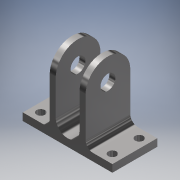
# Autodesk Inventor part: Custom Pneumatic Support
Saved by Autodesk Inventor 2019.4 (Build 234330000, 330)
## iProperties
Created: 2020-01-02
Part Number: Custom Pneumatic Support
Material: Stainless Steel
Document SubType Name: Modeling
Designer: Mark
Mass: 154.479 g
Surface Area: 101.01 cm^2
Volume: 19.3099 cm^3
Density: 8 g/cm^3
Appearance: Semi-Polished
Author: Mark
Autodesk Inventor part; units mm, degrees
ref_plane "YZ Plane" through (0, 0, 0) normal (1, 0, 0) x (0, 1, 0)
ref_plane "XZ Plane" through (0, 0, 0) normal (0, 1, 0) x (-1, 0, 0)
ref_plane "XY Plane" through (0, 0, 0) normal (0, 0, 1) x (1, 0, 0)
sketch "Sketch1" plane through (0, 0, 0) normal (0, 1, 0) x (-1, 0, 0)
  line L0 (-30, 15) -> (30, 15)
  line L1 (30, 15) -> (30, -15)
  line L2 (30, -15) -> (-30, -15)
  line L3 (-30, -15) -> (-30, 15)
  line L4 (-30, 15) -> (30, -15) construction
  line L5 (30, 15) -> (-30, -15) construction
  circle A0 centre (24, -9) radius 2.75
  circle A1 centre (24, 9) radius 2.75
  circle A2 centre (-24, 9) radius 2.75
  circle A3 centre (-24, -9) radius 2.75
  point P0 (0, 0)
  dimension "d0" = 60
  dimension "d1" = 30
  dimension "d2" = 5.5
  dimension "d3" = 5.5
  dimension "d4" = 5.5
  dimension "d5" = 5.5
  dimension "d6" = 6
  dimension "d7" = 6
  dimension "d8" = 6
  dimension "d9" = 6
  dimension "d10" = 6
  dimension "d11" = 6
  dimension "d12" = 6
  dimension "d13" = 6
  constraints: 12 end point, 4 centre point, 2 midpoint, 2 parallel, 1 horizontal, 1 perpendicular
  measures "d0" distance of L1.end L2.end
  measures "d1" distance of L0.end L1.end
  measures "d2" diameter of A0
  measures "d3" diameter of A1
  measures "d4" diameter of A2
  measures "d5" diameter of A3
  measures "d6" distance from line of L3 A3.centre
  measures "d7" distance from line of L3 A2.centre
  measures "d8" distance from line of L2 A3.centre
  measures "d9" distance from line of L0 A2.centre
  measures "d10" distance from line of L2 A0.centre
  measures "d11" distance from line of A1.centre L0
  measures "d12" distance from line of L1 A1.centre
  measures "d13" distance from line of L1 A0.centre
extrude "Extrusion1" add sketch "Sketch1" along normal blind 5
sketch "Sketch2" plane through (0, 5, 0) normal (0, 1, 0) x (1, 0, 0)
  line L0 (8, -15) -> (-8, -15)
  line L1 (-8, -15) -> (-8, 15)
  line L2 (-8, 15) -> (8, 15)
  line L3 (8, 15) -> (8, -15)
  line L4 (8, -15) -> (-8, 15) construction
  line L5 (-8, -15) -> (8, 15) construction
  line L6 (-8, 15) -> (-12, 15)
  line L7 (-12, 15) -> (-12, -15)
  line L8 (-12, -15) -> (-8, -15)
  line L9 (-8, -15) -> (-8, 15)
  line L10 (8, -15) -> (12, -15)
  line L11 (12, -15) -> (12, 15)
  line L12 (12, 15) -> (8, 15)
  line L13 (8, 15) -> (8, -15)
  point P0 (0, 0)
  dimension "d16" = 16
  dimension "d17" = 30
  dimension "d18" = 4
  dimension "d19" = 30
  dimension "d20" = 4
  constraints: 28 end point, 6 parallel, 3 horizontal, 3 perpendicular, 2 midpoint, 1 point on line
  measures "d16" distance of L1.end L2.end
  measures "d17" distance of L0.end L1.end
  measures "d18" distance of L8.end L7.end
  measures "d19" distance of L7.end L6.end
  measures "d20" distance of L12.end L11.end
extrude "Extrusion2" add sketch "Sketch2" along normal blind 46 contours L3 L12 L11 L10 | L8 L7 L6 L1
sketch "Sketch3" plane through (12, 5, 15) normal (1, 0, 0) x (0, 0, -1)
  circle A0 centre (15, 31) radius 5
  line L0 (30, 0) -> (30, 46) projected
  line L1 (30, -5) -> (0, -5) projected
  point P0 (15, -5)
  dimension "d23" = 10
  dimension "d24" = 15
  dimension "d25" = 36
  constraints: 1 centre point
  measures "d23" diameter of A0
  measures "d24" distance from line of L0 A0.centre
  measures "d25" distance from line of L1 A0.centre
extrude "Extrusion3" cut sketch "Sketch3" against normal blind 40
fillet "Fillet1" radius 15 4 edges at (10, 51, 15) (10, 51, -15) (-10, 51, -15) (-10, 51, 15)
fillet "Fillet2" radius 5 2 edges at (12, 5, 0) (-12, 5, 0)
fillet "Fillet3" radius 8 2 edges at (-8, 5, 0) (8, 5, 0)
body "Solid1"
